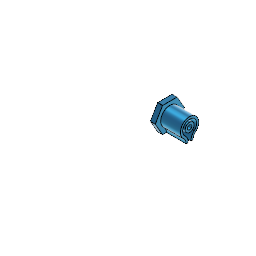
Z Belt Anchor Top Lock_2x (Autodesk Fusion 360 design; units mm, degrees)
Autodesk Fusion 360 part; units mm, degrees
sketch "Sketch2" plane through (-20, 0, 0) normal (-1, 0, 0) x (0, -1, 0)
  line L0 (-64, 10) -> (-54, 0)
  line L1 (-54, 0) -> (-42, 0)
  line L2 (-33.5, 0) -> (-32, 3)
  line L3 (-32, 3) -> (-30.5, 0)
  line L4 (-30.5, 0) -> (-10, 0)
  line L5 (-10, 0) -> (0, 10)
  line L6 (0, 10) -> (0, 24)
  line L7 (0, 24) -> (-30.5, 24)
  line L8 (-30.5, 24) -> (-32, 21)
  line L9 (-32, 21) -> (-33.5, 24)
  line L10 (-33.5, 24) -> (-64, 24)
  line L11 (-64, 24) -> (-64, 10)
  line L12 (-42, 0) -> (-36, 0)
  circle A0 centre (-19.25, 10) radius 5 construction
  circle A1 centre (-19.25, 10) radius 2.75
  arc A2 (-42, 0) -> (-43.974, 4.3867) centre (-47.8611, 0) ccw
  arc A3 (-34.026, 4.3867) -> (-43.974, 4.3867) centre (-39, 10) ccw
  arc A4 (-34.026, 4.3867) -> (-36, 0) centre (-30.1389, 0) ccw
  line L13 (-36, 0) -> (-33.5, 0)
  line L14 (-64, 10) -> (-54, 0)
  line L15 (-54, 0) -> (-42, 0)
  arc A5 (-42, 0) -> (-43.974, 4.3867) centre (-47.8611, 0) ccw
  arc A6 (-34.026, 4.3867) -> (-43.974, 4.3867) centre (-39, 10) ccw
  arc A7 (-34.026, 4.3867) -> (-36, 0) centre (-30.1389, 0) ccw
  line L16 (-36, 0) -> (-33.5, 0)
  line L17 (-33.5, 0) -> (-32, 3)
  line L18 (-32, 3) -> (-30.5, 0)
  line L19 (-30.5, 0) -> (-10, 0)
  line L20 (-10, 0) -> (0, 10)
  line L21 (0, 10) -> (0, 24)
  line L22 (0, 24) -> (-30.5, 24)
  line L23 (-30.5, 24) -> (-32, 21)
  line L24 (-32, 21) -> (-33.5, 24)
  line L25 (-33.5, 24) -> (-64, 24)
  line L26 (-64, 24) -> (-64, 10)
  circle A8 centre (-19.25, 10) radius 2.75
  arc A9 (-42, 0) -> (-43.974, 4.3867) centre (-47.8611, 0) ccw
  arc A10 (-34.026, 4.3867) -> (-36, 0) centre (-30.1389, 0) ccw
  arc A11 (-34.026, 4.3867) -> (-43.974, 4.3867) centre (-39, 10) ccw
  circle A12 centre (-39, 10) radius 1.5
  line L27 (-64, 10) -> (-54, 0)
  line L28 (-54, 0) -> (-49.5, 0)
  line L29 (-49.5, 0) -> (-49.5, 20)
  line L30 (-49.5, 20) -> (-64, 20)
  line L31 (-64, 20) -> (-64, 10)
  circle A13 centre (-39, 10) radius 5.5
  circle A14 centre (-39, 10) radius 3.5
  arc A15 (-35.3524, 5.8836) -> (-38, 0) centre (-30.1389, 0) ccw
  arc A16 (-40, 0) -> (-42.6476, 5.8836) centre (-47.8611, 0) ccw
  dimension "d442" = 0
  dimension "d443" = 0
  dimension "d444" = 0
  dimension "d445" = 0
  dimension "d631" = 10
  dimension "d757" = 0
  dimension "d758" = 0
  dimension "d759" = 0
  dimension "d760" = 0
  dimension "d931" = 0
  dimension "d932" = 0
  dimension "d933" = 0
  dimension "d934" = 0
  dimension "d939" = 0
  dimension "d940" = 0
  dimension "d941" = 0
  dimension "d942" = 0
  measures "d631" diameter of A0
extrude "Extrude5" add sketch "Sketch2" against normal blind 15.5 contours L12 A2 A3 A4 A5 A6 A7 A9 A10 A11 A13 A15 A16 | A14 makes body 1 at (-9.6667, 41.3402, 17.1256) makes body 2 at (-9.6667, 35.5044, 9.8255)
extrude "Extrude3" add sketch "Sketch2" against normal blind 4.5 contours L12 A2 A3 A4 A5 A6 A7 A9 A10 A11 A13 A15 A16 | L12 A13 A15 A16 | A13 | A14 bodies 1 2
move_face "OffsetFaces2" offset -0.25 1 faces at (-9.6667, 39.6843, 8.6652) on bodies 1
move_face "OffsetFaces3" offset -0.25 1 faces at (-9.6667, 44.242, 4.6361) on bodies 1
sketch "Sketch3" plane through (-20, 0, 0) normal (-1, 0, 0) x (0, -1, 0)
  circle A0 centre (-39, 10) radius 1.75
  circle A1 centre (-39, 10) radius 10
  arc A2 (-34.026, 4.3867) -> (-43.974, 4.3867) centre (-39, 10) ccw
  line L0 (-33.2265, 0) -> (-27.453, 10)
  line L1 (-27.453, 10) -> (-33.2265, 20)
  line L2 (-33.2265, 20) -> (-44.7735, 20)
  line L3 (-44.7735, 20) -> (-50.547, 10)
  line L4 (-50.547, 10) -> (-44.7735, 0)
  line L5 (-44.7735, 0) -> (-33.2265, 0)
  dimension "d922" = 2.5
  dimension "d923" = 20
  measures "d922" distance of A1 A2
  measures "d923" diameter of A1
extrude "Extrude6" add sketch "Sketch3" along normal blind 4 bodies 1
named bodies: "Z Belt Top Anchor Lock"
